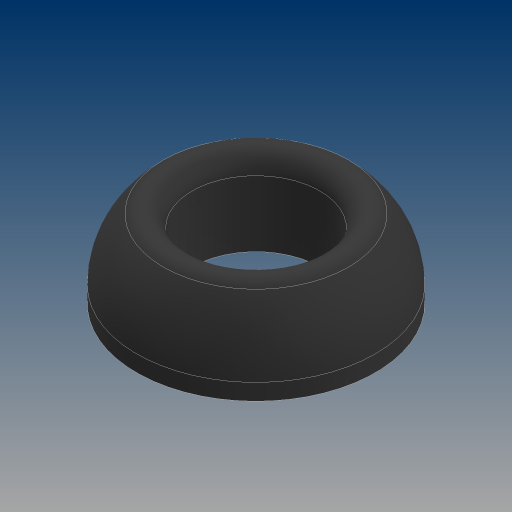
# Autodesk Inventor part: ELEV_010_BOLTCOVER2
Saved by Autodesk Inventor 2024.3 (Build 283343000, 343)
## iProperties
Created: 2024-11-25
Part Number: ELEV_010_BOLTCOVER2
Material: Rubber
Document SubType Name: Modeling
Designer: Kenji
Density: 0.93 g/cm^3
Appearance: Rubber - Black
Author: Kenji
Autodesk Inventor part; units mm, degrees
ref_plane "YZ Plane" through (0, 0, 0) normal (1, 0, 0) x (0, 1, 0)
ref_plane "XZ Plane" through (0, 0, 0) normal (0, 1, 0) x (-1, 0, 0)
ref_plane "XY Plane" through (0, 0, 0) normal (0, 0, 1) x (1, 0, 0)
sketch "Sketch1" plane through (0, 0, 0) normal (0, 1, 0) x (-1, 0, 0)
  circle A0 centre (0, 0) radius 2.3813
  circle A1 centre (0, 0) radius 4.445
  dimension "d0" = 4.7625
  dimension "d1" = 8.89
  constraints: 2 centre point, 2 coincident
  measures "d0" diameter of A0
  measures "d1" diameter of A1
extrude "Extrusion1" add sketch "Sketch1" along normal blind 3.5814
fillet "Fillet1" radius 3.175 1 edges at (4.445, 3.5814, 0)
fillet "Fillet2" radius 0.635 1 edges at (2.3813, 3.5814, 0)
body "Solid1"
